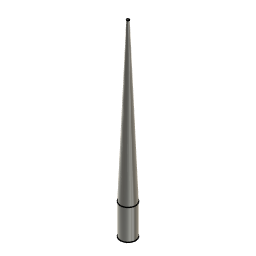
spring_tip_holder_assembly v11 (Autodesk Fusion 360 archive; units mm, degrees)
design "single tip press fit"
Autodesk Fusion 360 part; units mm, degrees
sketch "Sketch1" plane through (0, 0, 0) normal (0, 0, 1) x (1, 0, 0)
  circle A0 centre (0, 0) radius 1.5875
  dimension "d1" = 3.175
  dimension "d6" = 0
  constraint coincident A0.centre origin
  measures "d1" diameter of A0
ref_plane "WorkPlane1" through (0, 0, 33.02) normal (0, 0, 1) x (1, 0, 0)
sketch "Sketch2" plane through (0, 0, 33.02) normal (0, 0, 1) x (1, 0, 0)
  circle A0 centre (0, 0) radius 0.254
  dimension "d3" = 0.508
  constraint coincident A0.centre origin
  measures "d3" diameter of A0
loft "Loft1" add profiles "Sketch1", "Sketch2" section 1 section 2
extrude "Extrude2" add 1 faces at (-0.3879, 0.3599, 0) along direction (0, 0, -1) blind 6.35
sketch "Sketch4" plane through (0, 0, 0) normal (0, 1, 0) x (1, 0, 0)
equation "d1 = ( 1 / 8 ) * 1 in"

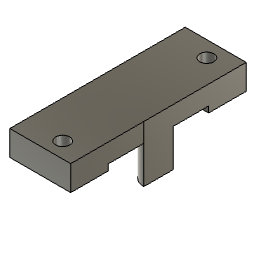
design "Screw Holder"
Autodesk Fusion 360 part; units mm, degrees
sketch "Sketch1" plane through (0, 0, 0) normal (0, 0, 1) x (1, 0, 0)
  line L0 (0, 2.9845) -> (0, -2.9845)
  arc A0 (0, 2.9845) -> (0, -2.9845) centre (0, 0) ccw
  dimension "d1" = 5.969
  constraint coincident A0.centre origin
  constraint vertical L0
  measures "d1" diameter of A0
extrude "Extrude1" add sketch "Sketch1" along normal blind 6.35 makes body 1
sketch "Sketch2" plane through (0, 0, 6.35) normal (0, 0, 1) x (-1, 0, 0)
  arc A0 (0, -2.9845) -> (0, 2.9845) centre (0, 0) ccw
  line L0 (0, 2.9845) -> (0, -2.9845)
  line L1 (15.24, -17.78) -> (0, -17.78)
  line L2 (0, -17.78) -> (0, 0)
  line L3 (0, 0) -> (15.24, 0) construction
  circle A1 centre (4.8006, -14.605) radius 1.4224
  circle A2 centre (4.8006, 14.605) radius 1.4224
  line L4 (0, 17.78) -> (0, 0)
  line L5 (15.24, 17.78) -> (0, 17.78)
  line L6 (15.24, -17.78) -> (15.24, 17.78)
  line L7 (0, -6.35) -> (0, 0)
  line L8 (0, -10.16) -> (8.89, -10.16)
  line L9 (11.43, -7.62) -> (11.43, 7.62)
  line L10 (8.89, 10.16) -> (0, 10.16)
  line L11 (2.9845, 0) -> (2.9845, -10.16) construction
  line L12 (2.9845, 0) -> (2.9845, 10.16) construction
  arc A3 (11.43, 7.62) -> (8.89, 10.16) centre (8.89, 7.62) ccw
  arc A4 (8.89, -10.16) -> (11.43, -7.62) centre (8.89, -7.62) ccw
  point P0 (11.43, -10.16)
  dimension "d5" = 17.78
  dimension "d12" = 2.8448
  dimension "d13" = 15.24
  dimension "d14" = 15.24
  dimension "d15" = 3.175
  dimension "d16" = 11.43
  dimension "d18" = 10.16
  dimension "d19" = 10.16
  dimension "d22" = 2.54
  dimension "d35" = 10.4394
  constraint horizontal L1
  constraint vertical L2
  constraint coincident A0.centre L2.end
  constraint symmetric L3 A1 A2
  constraint symmetric A0.centre L3 L2.end
  constraint symmetric L1.start L3 L5.start
  constraint symmetric L1.end L3 L4.start
  constraint midpoint L3.end L6
  constraint coincident L2 L7.start
  constraint coincident L4 A0.centre
  constraint coincident L7 L8.start
  constraint coincident L2 L8.start
  constraint perpendicular L8 L9
  constraint coincident L7 L10.end
  constraint perpendicular L7 L10
  constraint parallel L7 L9
  constraint midpoint A0 L11.start
  constraint coincident L8 L11.end
  constraint tangent A0 L11
  constraint vertical L11
  constraint coincident L10 L12.end
  constraint perpendicular L10 L12
  constraint tangent L9 A3
  constraint tangent L10 A3
  constraint coincident P0 L8
  constraint coincident P0 L9
  constraint tangent L8 A4
  constraint tangent L9 A4
  constraint equal A3 A4
  measures "d5" distance of A0.centre L1.end
  measures "d12" diameter of A1
  measures "d13" distance of L1.start L1.end
  measures "d14" horizontal distance of L4.start L5.start
  measures "d15" distance of L1 A1.centre
  measures "d16" distance of L8.start P0
  measures "d18" distance of L11.start L11.end
  measures "d19" distance of L11.start L12.end
  measures "d22" radius of A3
  measures "d35" distance of A2.centre L6
extrude "Extrude2" add sketch "Sketch2" along normal blind 5.08 separate body contours A0 L2 L4 L7 L8 L9 L10 A3 A4 | L1 L2 L4 L5 L6 L8 L9 L10 A3 A4 makes body 2
extrude "Extrude3" add 1 faces at (-0.8616, -0.4974, 6.35) along direction (0, 0, 1) blind 5.08 on bodies 1 bodies 1 2
extrude "Extrude4" cut sketch "Sketch2" along normal blind 1.2383 contours A0 L2 L4 L7 L8 L9 L10 A3 A4 bodies 1
extrude "Extrude5" cut 1 faces at (-15.24, 5.9267, 8.0433) along direction (1, 0, 0) blind 2.8956 on bodies 1 bodies 1
equation "d5 = ( 1.4 / 2 ) * 1 in"

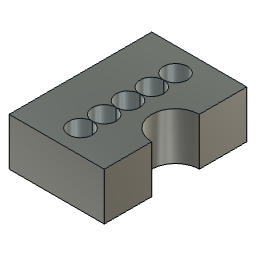
design "base for 5 tips press fit"
Autodesk Fusion 360 part; units mm, degrees
sketch "Sketch1" plane through (0, 0, 0) normal (0, 0, 1) x (1, 0, 0)
  line L0 (-6.35, 9.525) -> (6.35, 9.525)
  line L1 (6.35, 9.525) -> (6.35, -9.525)
  line L2 (6.35, -9.525) -> (-6.35, -9.525)
  line L3 (-6.35, -9.525) -> (-6.35, 9.525)
  line L4 (0, 0) -> (0, 3.175) construction
  line L5 (0, 3.175) -> (0, 6.35) construction
  line L6 (0, 0) -> (0, -3.175) construction
  line L7 (0, -3.175) -> (0, -6.35) construction
  circle A0 centre (0, 6.35) radius 1.5875
  circle A1 centre (0, 3.175) radius 1.5875
  circle A2 centre (0, 0) radius 1.5875
  circle A3 centre (0, -3.175) radius 1.5875
  circle A4 centre (0, -6.35) radius 1.5875
  arc A5 (6.35, 3.175) -> (6.35, -3.175) centre (6.35, 0) ccw
  dimension "d3" = 12.7
  dimension "d4" = 19.05
  dimension "d5" = 3.175
  dimension "d6" = 3.175
  dimension "d7" = 3.175
  dimension "d8" = 3.175
  dimension "d9" = 3.175
  dimension "d10" = 3.175
  dimension "d11" = 3.175
  dimension "d12" = 3.175
  dimension "d13" = 3.175
  dimension "d21" = 6.35
  constraint horizontal L0
  constraint vertical L1
  constraint horizontal L2
  constraint vertical L3
  constraint coincident L4.start L6.start
  constraint vertical L4
  constraint parallel L4 L5
  constraint parallel L4 L6
  constraint parallel L6 L7
  constraint coincident L5.end A0.centre
  constraint coincident L4.end L5.start
  constraint coincident L6.end L7.start
  constraint coincident L7.end A4.centre
  constraint midpoint L1 A5.centre
  constraint coincident L1 A5.end
  constraint coincident L1 A5.start
  measures "d3" distance of L0.start L0.end
  measures "d4" distance of L0.start L2.end
  measures "d5" distance of L4.start L4.end
  measures "d6" distance of L4.end L5.end
  measures "d7" distance of L4.start L6.end
  measures "d8" distance of L6.end L7.end
  measures "d9" diameter of A0
  measures "d10" diameter of A1
  measures "d11" diameter of A2
  measures "d12" diameter of A3
  measures "d13" diameter of A4
  measures "d21" diameter of A5
extrude "Extrude1" add sketch "Sketch1" along normal blind 6.35 contours L0 L1 L2 L3 A5
sketch "Sketch2" plane through (0, 0, 6.35) normal (0, 0, 1) x (-1, 0, 0)
  circle A0 centre (0, 6.35) radius 1.5875
  circle A1 centre (0, -6.35) radius 1.5875
  line L0 (6.35, 9.525) -> (-6.35, 9.525)
  line L1 (-6.35, -3.175) -> (-6.35, -9.525)
  line L2 (-6.35, -9.525) -> (6.35, -9.525)
  line L3 (6.35, -9.525) -> (6.35, 9.525)
  arc A2 (1.905, 6.35) -> (-1.905, 6.35) centre (0, 6.35) ccw
  arc A3 (-1.905, -6.35) -> (1.905, -6.35) centre (0, -6.35) ccw
  circle A4 centre (0, -3.175) radius 1.5875
  arc A5 (0, -1.5875) -> (0, 1.5875) centre (0, 0) ccw
  arc A6 (0, 1.5875) -> (0, 4.7625) centre (0, 3.175) ccw
  arc A7 (0, -1.5875) -> (0, -4.7625) centre (0, -3.175) ccw
  arc A8 (0, 1.5875) -> (0, -1.5875) centre (0, 0) ccw
  arc A9 (0, 4.7625) -> (0, 1.5875) centre (0, 3.175) ccw
  line L4 (-6.35, 9.525) -> (-6.35, 3.175)
  arc A10 (-6.35, -3.175) -> (-6.35, 3.175) centre (-6.35, 0) ccw
  dimension "d17" = 3.81
  dimension "d18" = 3.81
  constraint concentric A0 A2
  constraint coincident L3 A2.start
  constraint concentric A1 A3
  measures "d17" diameter of A2
  measures "d18" diameter of A3
sketch "Sketch3" plane through (0, 0, 6.35) normal (0, 0, 1) x (-1, 0, 0)
  circle A0 centre (0, 6.35) radius 1.5875
  arc A1 (0, 1.5875) -> (0, 4.7625) centre (0, 3.175) ccw
  arc A2 (0, -1.5875) -> (0, 1.5875) centre (0, 0) ccw
  arc A3 (0, -4.7625) -> (0, -1.5875) centre (0, -3.175) ccw
  circle A4 centre (0, -6.35) radius 1.5875
  arc A5 (0, -1.5875) -> (0, -4.7625) centre (0, -3.175) ccw
  arc A6 (0, 1.5875) -> (0, -1.5875) centre (0, 0) ccw
  arc A7 (0, 4.7625) -> (0, 1.5875) centre (0, 3.175) ccw
  line L0 (-6.35, -3.175) -> (-6.35, -9.525)
  line L1 (-6.35, -9.525) -> (6.35, -9.525)
  line L2 (6.35, -9.525) -> (6.35, 9.525)
  line L3 (6.35, 9.525) -> (-6.35, 9.525)
  line L4 (-6.35, 9.525) -> (-6.35, 3.175)
  arc A8 (-6.35, -3.175) -> (-6.35, 3.175) centre (-6.35, 0) ccw
sketch "Sketch4" plane through (-6.35, 0, 0) normal (-1, 0, 0) x (0, -1, 0)
  line L0 (-9.525, 0) -> (9.525, 0)
  line L1 (9.525, 0) -> (9.525, 6.35)
  line L2 (9.525, 6.35) -> (-9.525, 6.35)
  line L3 (-9.525, 6.35) -> (-9.525, 0)
  line L4 (0, 0) -> (0, 3.175) construction
  circle A0 centre (0, 3.175) radius 1.905
  dimension "d22" = 3.175
  dimension "d23" = 3.81
  constraint coincident L4.start origin
  constraint perpendicular L0 L4
  constraint coincident L4.end A0.centre
  measures "d22" distance of L4.start L4.end
  measures "d23" diameter of A0
extrude "Extrude3" cut sketch "Sketch4" against normal blind 3.81 contours A0
thread "Thread1" "ANSI Unified Screw Threads 0.164(#8) 8-32 UNC 3B" major diameter 4.1656 minor diameter 3.4163 pitch 0.7937 angle 60 resizes the face on face at (-3.81, -1.8955, 2.9853)
equation "d9 = ( 1 / 8 ) * 1 in"
equation "d10 = ( 1 / 8 ) * 1 in"
equation "d11 = ( 1 / 8 ) * 1 in"
equation "d13 = ( 1 / 8 ) * 1 in"
equation "d21 = ( 1 / 4 ) * 1 in"
equation "d22 = ( 1 / 8 ) * 1 in"

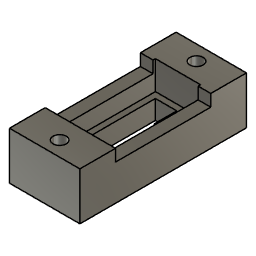
design "connection_PS_top"
Autodesk Fusion 360 part; units mm, degrees
sketch "Sketch1" plane through (0, 0, 0) normal (0, 0, 1) x (1, 0, 0)
  circle A0 centre (14.6002, 31.1293) radius 1.4224
  line L0 (22.0628, -1.2359) -> (22.0962, 34.2883)
  line L1 (22.0628, -1.2359) -> (3.0128, -1.2359)
  circle A1 centre (14.5728, 1.9372) radius 1.4224
  line L2 (22.0962, 34.2883) -> (3.0462, 34.3241)
  line L3 (19.391, 6.3752) -> (6.183, 6.3752)
  line L4 (6.183, 6.3752) -> (6.183, 27.2032)
  line L5 (6.183, 27.2032) -> (19.391, 27.2032)
  line L6 (19.391, 27.2032) -> (19.391, 6.3752)
  line L7 (19.391, 6.3752) -> (6.183, 27.2032) construction
  line L8 (6.183, 6.3752) -> (19.391, 27.2032) construction
  line L9 (3.0462, 34.3241) -> (3.0128, -1.2359)
  point P0 (3.0128, 16.5441)
  point P1 (12.787, 16.7892)
  dimension "d1" = 17.78
  dimension "d3" = 2.8448
  dimension "d14" = 20.828
  dimension "d16" = 13.208
  dimension "d17" = 19.05
  dimension "d61" = 7.493
  dimension "d62" = 7.493
  constraint horizontal L1
  constraint horizontal L3
  constraint perpendicular L3 L4
  constraint parallel L3 L5
  constraint parallel L4 L6
  constraint coincident L7 P1
  constraint coincident L8 P1
  measures "d1" distance of L1.end P0
  measures "d3" diameter of A1
  measures "d14" distance of L3 L5
  measures "d16" distance of L4.end L5.end
  measures "d17" distance of L0.end L2.end
  measures "d61" distance of A1.centre L0
  measures "d62" distance of A0.centre L0
extrude "Extrude3" add sketch "Sketch1" along normal blind 10.16
sketch "Sketch5" plane through (0, 0, 0) normal (0, 0, -1) x (1, 0, 0)
  circle A0 centre (14.6002, -31.1293) radius 1.4224
  line L0 (19.391, -27.2032) -> (6.183, -27.2032)
  line L1 (6.183, -27.2032) -> (6.183, -6.3752)
  line L2 (6.183, -6.3752) -> (19.391, -6.3752)
  line L3 (19.391, -6.3752) -> (19.391, -27.2032)
  circle A1 centre (14.5728, -1.9372) radius 1.4224
  line L4 (22.0962, -34.2883) -> (22.0628, 1.2359)
  line L5 (22.0628, 1.2359) -> (3.0128, 1.2359)
  line L6 (3.0128, 1.2359) -> (3.0462, -34.3241)
  line L7 (3.0462, -34.3241) -> (22.0962, -34.2883)
  line L8 (19.391, -27.2032) -> (15.581, -27.2032)
  line L9 (15.581, -27.2032) -> (15.581, -6.3732)
  line L10 (15.581, -6.3732) -> (19.391, -6.3732)
  line L11 (19.391, -6.3732) -> (19.391, -27.2032)
  line L12 (15.3014, -12.0362) -> (15.4278, -21.1048)
  line L13 (15.4278, -21.1048) -> (19.391, -21.1048)
  line L14 (19.391, -16.7892) -> (15.3014, -12.0362) construction
  line L15 (15.4278, -21.1048) -> (19.391, -16.7892) construction
  line L16 (19.391, -12.0293) -> (15.3014, -12.0362)
  line L17 (6.183, -27.2032) -> (8.723, -27.2032)
  line L18 (8.723, -27.2032) -> (8.723, -6.3752)
  line L19 (8.723, -6.3752) -> (6.183, -6.3752)
  line L20 (6.183, -6.3752) -> (6.183, -27.2032)
  dimension "d31" = 3.81
  dimension "d36" = 2.54
  constraint horizontal L8
  constraint vertical L9
  constraint horizontal L10
  constraint vertical L11
  constraint coincident L0.start L3.end
  constraint horizontal L13
  constraint midpoint L3 L14.start
  constraint coincident L3 L13.end
  constraint coincident L3 L16.start
  constraint horizontal L17
  constraint vertical L18
  constraint horizontal L19
  constraint vertical L20
  constraint coincident L2 L18.end
  constraint coincident L0.end L1.start
  measures "d31" distance of L0.start L8.end
  measures "d36" distance of L0.end L17.end
extrude "Extrude7" add sketch "Sketch5" against normal blind 4.064 contours L0 L3 L8 L9 L11 L13 | L0 L1 L2 L17 L18 L19 L20 | L2 L3 L9 L10 L11 L16
sketch "Sketch7" plane through (3.0139, -0.0028, 0) normal (-1, 0.000941, 0) x (-0.000941, -1, 0)
  line L0 (-34.327, 0) -> (1.233, 0)
  line L1 (1.233, 0) -> (1.233, 10.16)
  line L2 (1.233, 10.16) -> (-34.327, 10.16)
  line L3 (-34.327, 10.16) -> (-34.327, 0)
  line L4 (-6.387, 7.62) -> (-26.707, 7.62)
  line L5 (-26.707, 7.62) -> (-26.707, 10.16)
  line L6 (-6.387, 10.16) -> (-6.387, 7.62)
  dimension "d65" = 20.32
  dimension "d66" = 7.62
  constraint horizontal L4
  constraint perpendicular L4 L5
  constraint parallel L5 L6
  constraint coincident L2 L5.end
  constraint coincident L2 L6.start
  measures "d65" distance of L4.start L4.end
  measures "d66" distance of L3 L5
extrude "Extrude8" cut sketch "Sketch7" against normal blind 33.02 contours L2 L4 L5 L6
extrude "Extrude9" add 1 faces at (6.183, 20.0932, 5.2493) along direction (1, 0, 0) blind 3.556
extrude "Extrude10" add 1 faces at (8.723, 20.2605, 1.3547) along direction (1, 0, 0) blind 2.286
sketch "Sketch8" plane through (0, 27.2032, 0) normal (0, -1, 0) x (1, 0, 0)
  line L0 (11.009, 4.064) -> (11.009, 0)
  line L1 (11.009, 0) -> (15.581, 0)
  line L2 (15.581, 0) -> (15.581, 4.064)
  line L3 (15.581, 4.064) -> (19.391, 4.064)
  line L4 (19.391, 4.064) -> (19.391, 10.16)
  line L5 (19.391, 10.16) -> (9.739, 10.16)
  line L6 (9.739, 10.16) -> (9.739, 4.064)
  line L7 (9.739, 4.064) -> (11.009, 4.064)
  line L8 (11.009, 4.064) -> (15.581, 4.064)
  line L9 (15.581, 4.064) -> (15.581, 0)
  line L10 (15.581, 0) -> (11.009, 0)
  line L11 (11.009, 0) -> (11.009, 4.064)
  constraint horizontal L8
  constraint vertical L9
  constraint horizontal L10
  constraint vertical L11
  constraint coincident L1.end L2.start
  constraint coincident L0.start L7.end
extrude "Extrude13" add sketch "Sketch8" along normal blind 1.27 contours L0 L1 L2 L8 L9 L10 L11
sketch "Sketch9" plane through (0, 6.3752, 0) normal (0, 1, 0) x (-1, 0, 0)
  line L0 (-11.009, 0) -> (-11.009, 4.064)
  line L1 (-11.009, 4.064) -> (-9.739, 4.064)
  line L2 (-9.739, 4.064) -> (-9.739, 10.16)
  line L3 (-9.739, 10.16) -> (-12.533, 10.16)
  line L4 (-19.391, 7.62) -> (-19.391, 4.064)
  line L5 (-19.391, 4.064) -> (-15.581, 4.064)
  line L6 (-15.581, 4.064) -> (-15.581, 0)
  line L7 (-15.581, 0) -> (-11.009, 0)
  line L8 (-15.581, 4.064) -> (-11.009, 4.064)
  line L9 (-11.009, 4.064) -> (-11.009, 0)
  line L10 (-11.009, 0) -> (-15.581, 0)
  line L11 (-15.581, 0) -> (-15.581, 4.064)
  line L12 (-12.533, 10.16) -> (-12.533, 7.62)
  line L13 (-12.533, 7.62) -> (-19.391, 7.62)
  dimension "d47" = -1.27
  constraint horizontal L8
  constraint vertical L9
  constraint horizontal L10
  constraint vertical L11
  constraint coincident L0.start L7.end
  constraint coincident L5.end L6.start
extrude "Extrude14" add sketch "Sketch9" along normal blind 1.27 contours L0 L6 L7 L8 L9 L10 L11
extrude "Extrude15" cut 1 faces at (3.0327, 19.9308, 2.54) along direction (1, -0.000941, 0) blind 3.81
extrude "Extrude16" cut 2 faces at (6.6143, 6.3807, 8.4667) (6.6143, 6.3809, 7.62) along direction (0.000941, 1, 0) blind 5.08
extrude "Extrude17" cut 2 faces at (6.8379, 14.8473, 2.54) (6.8299, 6.3809, 9.3133) along direction (1, -0.000941, 0) blind 0.2032
extrude "Extrude18" cut 1 faces at (6.9654, 6.381, 9.3133) along direction (0.000941, 1, 0) blind 3.556
